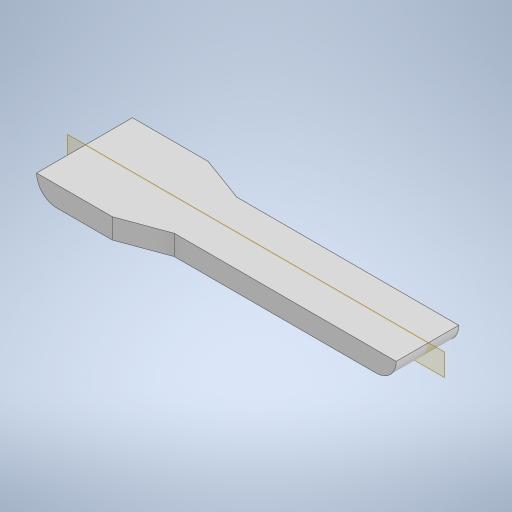
# Autodesk Inventor part: Arm_1D
Saved by Autodesk Inventor 2023 (Build 270158000, 158)
## iProperties
Created: 2024-07-29
Part Number: Arm_1D
Material: Generic
Document SubType Name: Modeling
Designer: Swoby
Density: 1 g/cm^3
Appearance: Default
Author: Swoby
Autodesk Inventor part; units mm, degrees
ref_plane "YZ Plane" through (0, 0, 0) normal (1, 0, 0) x (0, 1, 0)
ref_plane "XZ Plane" through (0, 0, 0) normal (0, 1, 0) x (-1, 0, 0)
sketch "Sketch1" plane through (0, 0, 0) normal (0, 0, 1) x (1, 0, 0)
  line L0 (-150, 0) -> (150, 0) construction
  line L1 (-150, -20) -> (150, -20)
  line L2 (150, 20) -> (-150, 20) construction
  arc A0 (-150, 20) -> (-170, 0) centre (-150, 0) ccw construction
  arc A1 (150, -20) -> (170, 0) centre (150, 0) ccw
  line L3 (0, 0) -> (300, 0) construction
  line L4 (-170, 0) -> (170, 0)
  arc A2 (-170, 0) -> (-150, -20) centre (-150, 0) ccw
  arc A3 (170, 0) -> (150, 20) centre (150, 0) ccw construction
  dimension "d0" = 150
  dimension "d2" = 40
  constraints: 12 end point, 8 point on circle, 8 tangent, 4 centre point, 2 horizontal, 2 parallel, 1 collinear, 1 midpoint, 1 point on line
  measures "d0" distance of L3.start L0.end
  measures "d2" diameter of A1
extrude "Extrusion1" add sketch "Sketch1" along normal mid plane 62
sketch "Sketch2" plane through (0, 0, 31) normal (0, 0, 1) x (1, 0, 0)
  line L0 (-150, -20) -> (150, -20) projected
  arc A0 (150, -20) -> (170, 0) centre (150, 0) ccw projected
  line L1 (170, 0) -> (-170, 0) projected
  arc A1 (-170, 0) -> (-150, -20) centre (-150, 0) ccw projected
  line L2 (-50, 0) -> (-50, -20)
  circle A2 centre (-150, 0) radius 20 construction
  point P0 (0, 0)
  dimension "d5" = 100
  constraints: 2 end point, 2 point on line, 1 coincident, 1 horizontal alignment, 1 perpendicular, 2 other
  measures "d5" distance from line of L2 A1.centre
extrude "Extrusion2" add sketch "Sketch2" along normal blind 16.5 and the other way blind 78.5 contours A1 L1 L2 L0
chamfer "Chamfer1" distance 45 distance2 16.5 1 edges at (-50, -10, 47.5) measured on face at (-50.5, -10, 47.5)
chamfer "Chamfer2" distance 45 distance2 16.5 1 edges at (-50, -10, -47.5) measured on face at (-50.5, -10, -47.5)
body "Solid1"
